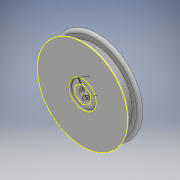
# Autodesk Inventor part: 모터기어
Saved by Autodesk Inventor 2018 (Build 220112000, 112)
## iProperties
Created: 2019-11-05
Part Number: 모터기어
Material: 일반
Document SubType Name: Modeling
Designer: LeeYounSeo
Density: 1 g/cm^3
Appearance: 기본값
Author: LeeYounSeo
Autodesk Inventor part; units mm, degrees
ref_plane "YZ Plane" through (0, 0, 0) normal (1, 0, 0) x (0, 1, 0)
ref_plane "XZ Plane" through (0, 0, 0) normal (0, 1, 0) x (-1, 0, 0)
ref_plane "XY Plane" through (0, 0, 0) normal (0, 0, 1) x (1, 0, 0)
sketch "스케치1" plane through (0, 0, 0) normal (0, 1, 0) x (-1, 0, 0)
  line L0 (2.4971, 1.4484) -> (2.5029, -1.4383)
  line L1 (2.5029, -1.4383) -> (0.0058, -2.8867)
  line L2 (0.0058, -2.8867) -> (-2.4971, -1.4484)
  line L3 (-2.4971, -1.4484) -> (-2.5029, 1.4383)
  line L4 (-2.5029, 1.4383) -> (-0.0058, 2.8867)
  line L5 (-0.0058, 2.8867) -> (2.4971, 1.4484)
  circle A0 centre (0, 0) radius 4.5
  circle A1 centre (0, 0) radius 15
  circle A2 centre (0, 0) radius 12.5
  dimension "d0" = 5
  dimension "d1" = 9
  dimension "d2" = 30
  dimension "d3" = 25
  constraints: 12 end point, 4 coincident, 3 centre point, 13 other
  measures "d0" distance between parallel lines of L3 L0
  measures "d1" diameter of A0
  measures "d2" diameter of A1
  measures "d3" diameter of A2
extrude "돌출1" add sketch "스케치1" along normal blind 5 contours A0
sketch "스케치2" plane through (0, 0, 0) normal (0, -1, 0) x (1, 0, 0)
  circle A0 centre (0, 0) radius 15
  circle A1 centre (0, 0) radius 4.5 projected
  dimension "d6" = 30
  constraints: 1 centre point, 1 coincident
  measures "d6" diameter of A0
extrude "돌출2" add sketch "스케치2" along normal blind 1
sketch "스케치3" plane through (0, 0, 0) normal (0, 1, 0) x (1, 0, 0)
  circle A0 centre (0, 0) radius 12.5
  circle A1 centre (0, 0) radius 4.5 projected
  dimension "d9" = 25
  constraints: 1 centre point, 1 coincident
  measures "d9" diameter of A0
extrude "돌출3" add sketch "스케치3" along normal blind 3
sketch "스케치4" plane through (0, 3, 0) normal (0, 1, 0) x (1, 0, 0)
  circle A0 centre (0, 0) radius 15
  circle A1 centre (0, 0) radius 4.5 projected
  dimension "d12" = 30
  constraints: 1 centre point, 1 coincident
  measures "d12" diameter of A0
extrude "돌출4" add sketch "스케치4" along normal blind 1
fillet "모깎기1" radius 1 2 edges at (-15, 0, 0) (-15, 3, 0)
sketch "스케치5" plane through (0, 0, 0) normal (0, -1, 0) x (1, 0, 0)
  circle A0 centre (0, 0) radius 4
  line L0 (-0.0058, -2.8867) -> (-2.5029, -1.4383) projected
  line L1 (-2.5029, -1.4383) -> (-2.4971, 1.4484) projected
  line L2 (-2.4971, 1.4484) -> (0.0058, 2.8867) projected
  line L3 (0.0058, 2.8867) -> (2.5029, 1.4383) projected
  line L4 (2.5029, 1.4383) -> (2.4971, -1.4484) projected
  line L5 (2.4971, -1.4484) -> (-0.0058, -2.8867) projected
  circle A1 centre (0, 0) radius 4.5 projected
  line L6 (-2.5029, -1.4383) -> (-2.4971, 1.4484) projected
  circle A2 centre (0, 0) radius 4.5 projected
  dimension "d16" = 8
  constraints: 1 centre point, 1 coincident
  measures "d16" diameter of A0
extrude "돌출5" add sketch "스케치5" along normal blind 0.5 contours A0 | L0 L1 L2 L3 L4 L5
sketch "스케치6" plane through (0, -0.5, 0) normal (0, -1, 0) x (1, 0, 0)
  circle A0 centre (0, 0) radius 1.6
  dimension "d19" = 3.2
  constraints: 1 centre point, 1 coincident
  measures "d19" diameter of A0
extrude "돌출6" cut sketch "스케치6" against normal blind 0.5
sketch "스케치7" plane through (0.0058, 0, 2.8867) normal (-0.5017425, 0, -0.8650171) x (-0.8650171, 0, 0.5017425)
  point P0 (-1.4434, 0)
sketch "스케치8" plane through (0, -1, 0) normal (0, -1, 0) x (1, 0, 0)
  point P0 (0, 0)
sketch "스케치9" plane through (0, -1, 0) normal (0, -1, 0) x (1, 0, 0)
  line L0 (-2.5029, -1.4383) -> (-0.0058, -2.8867) projected
  line L1 (-0.0058, -2.8867) -> (2.4971, -1.4484) projected
  line L2 (2.4971, -1.4484) -> (2.5029, 1.4383) projected
  line L3 (2.5029, 1.4383) -> (0.0058, 2.8867) projected
  line L4 (0.0058, 2.8867) -> (-2.4971, 1.4484) projected
  line L5 (-2.4971, 1.4484) -> (-2.5029, -1.4383) projected
  circle A0 centre (0, 0) radius 4.5 projected
  circle A1 centre (0, 0) radius 4.5 projected
  circle A2 centre (0, 0) radius 15 projected
  circle A3 centre (0, 0) radius 4.5 projected
move faces "이동1" translate (0, -0.5, 0) faces at (-3.1667, 5, 0.0034) (-4.4417, 4.3333, -0.7219)
move faces "이동2" translate (0, -0.5, 0) faces at (-3.1667, 4.5, 0.0034)
sketch "스케치10" plane through (0.0058, 0, 2.8867) normal (-0.5017425, 0, -0.8650171) x (-0.8650171, 0, 0.5017425)
  point P0 (-1.4434, 0)
sketch "스케치11" plane through (0, 4, 0) normal (0, 1, 0) x (1, 0, 0)
  line L0 (-0.0058, 2.8867) -> (2.4971, 1.4484) projected
  line L1 (0.0058, -2.8867) -> (-2.4971, -1.4484) projected
  point P0 (0, 0)
  dimension "d28" = 5
  measures "d28" distance between parallel lines of L0 L1
